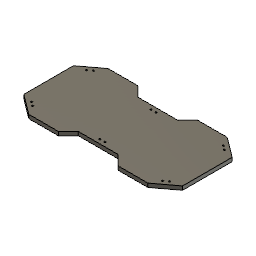
Body Top (Autodesk Fusion 360 design; units mm, degrees)
Autodesk Fusion 360 part; units mm, degrees
sketch "Sketch1" plane through (0, 0, 0) normal (0, 1, 0) x (1, 0, 0)
  line L0 (-160, -80) -> (160, -80)
  line L1 (160, -80) -> (160, 80)
  line L2 (160, 80) -> (-160, 80)
  line L3 (-160, 80) -> (-160, -80)
  line L4 (-160, -80) -> (160, 80) construction
  line L5 (160, -80) -> (-160, 80) construction
  line L6 (-160, -50) -> (-120, -80)
  line L7 (120, -80) -> (160, -50)
  line L8 (160, 50) -> (120, 80)
  line L9 (-120, 80) -> (-160, 50)
  line L10 (-120, -80) -> (-60, -80)
  line L11 (-40, -60) -> (-60, -80)
  line L12 (60, -80) -> (40, -60)
  line L13 (40, -60) -> (-40, -60)
  line L14 (-40, 60) -> (-60, 80)
  line L15 (-40, 60) -> (40, 60)
  line L16 (40, 60) -> (60, 80)
  dimension "d1" = 320
  dimension "d2" = 160
  constraint horizontal L0
  constraint perpendicular L0 L1
  constraint parallel L0 L2
  constraint parallel L1 L3
  constraint coincident L4 origin
  constraint coincident L5 origin
  constraint coincident L3 L6.start
  constraint coincident L0 L6.end
  constraint coincident L0 L7.start
  constraint coincident L1 L7.end
  constraint coincident L1 L8.start
  constraint coincident L2 L8.end
  constraint parallel L6 L8
  constraint coincident L2 L9.start
  constraint coincident L3 L9.end
  constraint parallel L7 L9
  constraint coincident L0 L10.end
  constraint coincident L0 L12.start
  constraint parallel L0 L13
  constraint coincident L2 L14.end
  constraint parallel L2 L15
  constraint coincident L2 L16.end
  constraint perpendicular L14 L16
  measures "d1" distance of L1.end L2.end
  measures "d2" distance of L0.end L1.end
extrude "Extrude1" add sketch "Sketch1" along normal blind 7.75 contours L0 L1 L2 L3 L6 L7 L8 L9 L10 L11 L12 L13 L14 L15 L16
sketch "Sketch2" plane through (0, 7.75, 0) normal (0, 1, 0) x (-1, 0, 0)
  line L0 (40, -60) -> (60, -80)
  line L1 (60, -80) -> (120, -80)
  line L2 (120, -80) -> (160, -50)
  line L3 (160, -50) -> (160, 50)
  line L4 (160, 50) -> (120, 80)
  line L5 (120, 80) -> (60, 80)
  line L6 (60, 80) -> (40, 60)
  line L7 (40, 60) -> (-40, 60)
  line L8 (-40, 60) -> (-60, 80)
  line L9 (-60, 80) -> (-120, 80)
  line L10 (-120, 80) -> (-160, 50)
  line L11 (-160, 50) -> (-160, -50)
  line L12 (-160, -50) -> (-120, -80)
  line L13 (-120, -80) -> (-60, -80)
  line L14 (-60, -80) -> (-40, -60)
  line L15 (-40, -60) -> (40, -60)
  circle A0 centre (-130.93, 61.24) radius 1.6
  circle A1 centre (-138.93, 55.24) radius 1.6
  circle A2 centre (-138.93, -55.24) radius 1.6
  circle A3 centre (-130.93, -61.24) radius 1.6
  circle A4 centre (5, -51.55) radius 1.6
  circle A5 centre (-5, -51.55) radius 1.6
  circle A6 centre (5, 51.55) radius 1.6
  circle A7 centre (-5, 51.55) radius 1.6
  circle A8 centre (138.93, 55.24) radius 1.6
  circle A9 centre (130.93, 61.24) radius 1.6
  circle A10 centre (130.93, -61.24) radius 1.6
  circle A11 centre (138.93, -55.24) radius 1.6
  dimension "d10" = 3.2
  dimension "d11" = 10
  dimension "d12" = 3.2
  dimension "d18" = 3.2
  dimension "d19" = 10
  dimension "d20" = 3.2
  dimension "d27" = 10
  dimension "d28" = 3.2
  dimension "d29" = 3.2
  dimension "d32" = 3.2
  dimension "d33" = 3.2
  dimension "d39" = 3.2
  dimension "d40" = 10
  dimension "d41" = 3.2
  dimension "d47" = 3.2
  dimension "d48" = 10
  dimension "d49" = 3.2
  measures "d10" diameter of A0
  measures "d11" distance of A0.centre A1.centre
  measures "d12" diameter of A1
  measures "d18" diameter of A2
  measures "d19" distance of A2.centre A3.centre
  measures "d20" diameter of A3
  measures "d27" distance of A4.centre A5.centre
  measures "d28" diameter of A4
  measures "d29" diameter of A5
  measures "d32" diameter of A6
  measures "d33" diameter of A7
  measures "d39" diameter of A8
  measures "d40" distance of A8.centre A9.centre
  measures "d41" diameter of A9
  measures "d47" diameter of A10
  measures "d48" distance of A10.centre A11.centre
  measures "d49" diameter of A11
extrude "Extrude2" cut sketch "Sketch2" against normal blind 35 contours A0 | A1 | A2 | A3 | A4 | A5 | A6 | A7 | A8 | A9 | A10 | A11
